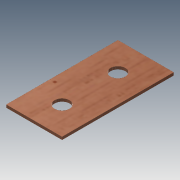
# Autodesk Inventor part: gabarito-travessa-60
Saved by Autodesk Inventor 2017 (Build 210142000, 142)
## iProperties
Created: 2018-08-29
Part Number: gabarito-travessa-60
Material: Wood (Oak)
Document SubType Name: Sheet Metal
Designer: Luiz Gustavo
Density: 0.76 g/cm^3
Sheet Metal Rule: Default_mm
Appearance: White Oak - Natural Medium Gloss
Author: Luiz Gustavo
Autodesk Inventor part; units mm, degrees
ref_plane "YZ Plane" through (0, 0, 0) normal (1, 0, 0) x (0, 1, 0)
ref_plane "XZ Plane" through (0, 0, 0) normal (0, 1, 0) x (-1, 0, 0)
ref_plane "XY Plane" through (0, 0, 0) normal (0, 0, 1) x (1, 0, 0)
sketch "Sketch1" plane through (0, 0, 0) normal (0, 0, 1) x (1, 0, 0)
  arc A0 (11.6513, 631.9608) -> (14.3394, 631.9567) centre (13, 635) ccw
  arc A1 (14.3394, 638.0433) -> (11.6606, 638.0433) centre (13, 635) ccw
  arc A2 (11.6513, 661.9608) -> (14.3394, 661.9567) centre (13, 665) ccw
  arc A3 (14.3394, 668.0433) -> (11.6606, 668.0433) centre (13, 665) ccw
  line L0 (25.9999, 620.0001) -> (17.4375, 620.0001)
  line L1 (0, 679.9999) -> (8.4375, 679.9999)
  circle A4 centre (13, 635) radius 4
  circle A5 centre (13, 665) radius 4
  line L2 (28, 620.0001) -> (-2, 620.0001)
  line L3 (-2, 620.0001) -> (-2, 679.9999)
  line L4 (-2, 679.9999) -> (28, 679.9999)
  line L5 (28, 679.9999) -> (28, 620.0001)
  line L6 (13, 620.0001) -> (13, 679.9999) construction
  point P0 (0, 0)
  dimension "d0" = 8
  dimension "d2" = 30
  measures "d0" diameter of A4
  measures "d2" distance of L3.end L4.end
extrude "Plate1" add sketch "Sketch1" along normal blind 1.5
equation "\"BendRadius\" = Thickness"
equation "\"BendReliefWidth\" = Thickness"
equation "\"BendReliefDepth\" = 0.5 * Thickness"
equation "\"CornerReliefSize\" = 4 * Thickness"
equation "\"MinimumRemnant\" = 2 * Thickness"
equation "\"TransitionRadius\" = BendRadius"
equation "\"JacobiRadiusSize\" = BendRadius"
equation "\"GapSize\" = Thickness"
equation "\"d3\" = BendRadius"
equation "\"Thickness\" = 1.5"
body "Solid1"
